Autodesk Inventor part; units mm, degrees
note: some values were not read from the file. Chosen so that the rebuilt part matches the saved one: direction of "Hole2".
(part 12 of 18)
  line L1418 (-102.9071, -28.2921) -> (-102.708, -28.311)
  line L1419 (-102.9072, -28.2921) -> (-102.9071, -28.2921)
  line L1420 (-102.7315, -28.5598) -> (-102.7316, -28.5598)
  line L1421 (-102.708, -28.311) -> (-102.7315, -28.5598)
  line L1422 (-102.8127, -27.2965) -> (-102.8128, -27.2965)
  line L1423 (-102.6136, -27.3154) -> (-102.8127, -27.2965)
  line L1424 (-102.59, -27.0665) -> (-102.6136, -27.3154)
  line L1425 (-102.5901, -27.0665) -> (-102.59, -27.0665)
  line L1426 (-102.9071, -28.2921) -> (-102.8127, -27.2965)
  line L1427 (-102.59, -27.0665) -> (-100.6985, -27.2458)
  line L1428 (-100.84, -28.7391) -> (-102.7315, -28.5598)
  line L1429 (-100.523, -27.5136) -> (-100.6173, -28.5091)
  line L1430 (-100.84, -28.7391) -> (-100.8164, -28.4902)
  line L1431 (-100.8164, -28.4902) -> (-100.6173, -28.5091)
  line L1432 (-100.6173, -28.5091) -> (-100.6174, -28.5091)
  line L1433 (-100.8401, -28.7391) -> (-100.84, -28.7391)
  line L1434 (-100.523, -27.5136) -> (-100.7221, -27.4947)
  line L1435 (-100.7221, -27.4947) -> (-100.6985, -27.2458)
  line L1436 (-102.4145, -27.3343) -> (-100.9212, -27.4758)
  line L1437 (-100.9212, -27.4758) -> (-101.0155, -28.4714)
  line L1438 (-101.0155, -28.4714) -> (-102.5088, -28.3298)
  line L1439 (-102.5088, -28.3298) -> (-102.4145, -27.3343)
  line L1440 (-101.1134, -27.6347) -> (-102.2557, -27.5265)
  line L1441 (-100.9212, -27.4758) -> (-101.1134, -27.6347)
  line L1442 (-102.4145, -27.3343) -> (-102.2557, -27.5265)
  line L1443 (-102.2557, -27.5265) -> (-102.3167, -28.1709)
  line L1444 (-102.5088, -28.3298) -> (-102.3167, -28.1709)
  line L1445 (-102.3167, -28.1709) -> (-101.1745, -28.2792)
  line L1446 (-101.0155, -28.4714) -> (-101.1745, -28.2792)
  line L1447 (-101.1745, -28.2792) -> (-101.1134, -27.6347)
  circle A31 centre (-101.9758, -27.8781) radius 0.1
  line L1448 (-101.8288, -28.0427) -> (-102.1512, -28.0122)
  line L1449 (-102.1512, -28.0122) -> (-102.1228, -27.7135)
  line L1450 (-102.1512, -28.0122) -> (-102.1229, -27.7135)
  line L1451 (-102.1228, -27.7135) -> (-101.8005, -27.7441)
  line L1452 (-101.8005, -27.7441) -> (-101.8288, -28.0427)
  line L1453 (-100.4365, -16.4719) -> (-100.4365, -16.671)
  line L1454 (-100.4365, -16.671) -> (-100.6865, -16.671)
  line L1455 (-99.4365, -16.671) -> (-99.4365, -16.4719)
  line L1456 (-99.1865, -16.671) -> (-99.4365, -16.671)
  line L1457 (-100.4365, -16.4719) -> (-99.4365, -16.4719)
  line L1458 (-99.1865, -16.671) -> (-99.1865, -18.4771)
  line L1459 (-100.6865, -18.4771) -> (-100.6865, -16.671)
  line L1460 (-99.4365, -16.8701) -> (-99.4365, -18.2782)
  line L1461 (-100.4365, -18.2782) -> (-100.4365, -16.8701)
  line L1462 (-100.4365, -16.8701) -> (-99.4365, -16.8701)
  line L1463 (-99.6129, -17.6207) -> (-99.6129, -17.14)
  line L1464 (-99.4365, -16.8701) -> (-99.6129, -17.14)
  line L1465 (-99.6129, -17.14) -> (-100.2602, -17.14)
  line L1466 (-100.4365, -16.8701) -> (-100.2602, -17.14)
  line L1467 (-100.2602, -17.14) -> (-100.2602, -17.6207)
  ellipse E657 centre (-99.9365, -17.4268) end of major axis (-99.8365, -17.4268) minor radius 0.0996
  ellipse E658 centre (-99.9365, -17.4315) end of major axis (-99.8365, -17.4315) minor radius 0.0996 (-100.0365, -17.4315) -> (-99.8365, -17.4315) ccw
  line L1468 (-100.0365, -17.4315) -> (-100.0365, -17.4268)
  line L1469 (-99.8365, -17.4315) -> (-99.8365, -17.4268)
  line L1470 (-100.0865, -17.5927) -> (-100.0865, -17.2703)
  line L1471 (-100.0865, -17.6115) -> (-100.0865, -17.5927)
  line L1472 (-100.0865, -17.2703) -> (-99.7865, -17.2703)
  line L1473 (-99.7865, -17.2703) -> (-99.7865, -17.5927)
  line L1474 (-99.7865, -17.6115) -> (-99.7865, -17.5927)
  line L1475 (-99.7865, -17.5927) -> (-100.0865, -17.5927)
  line L1476 (-99.7865, -17.6115) -> (-100.0865, -17.6115)
  line L1477 (-98.1515, -27.0495) -> (-97.9515, -27.0495)
  line L1478 (-98.1515, -27.08) -> (-98.1515, -27.0495)
  line L1479 (-97.9515, -27.2984) -> (-97.9515, -27.3284)
  line L1480 (-97.9515, -27.0495) -> (-97.9515, -27.2984)
  line L1481 (-97.9515, -26.054) -> (-98.1515, -26.054)
  line L1482 (-97.9515, -25.8051) -> (-97.9515, -26.054)
  line L1483 (-98.1515, -27.0495) -> (-98.1515, -26.054)
  line L1484 (-97.9515, -25.8051) -> (-96.0515, -25.8051)
  line L1485 (-96.0515, -27.2984) -> (-97.9515, -27.2984)
  line L1486 (-95.8515, -26.054) -> (-95.8515, -27.0495)
  line L1487 (-96.0515, -27.2984) -> (-96.0515, -27.0495)
  line L1488 (-96.0515, -27.0495) -> (-95.8515, -27.0495)
  line L1489 (-95.8515, -27.0495) -> (-95.8515, -27.08)
  line L1490 (-96.0515, -27.3284) -> (-96.0515, -27.2984)
  line L1491 (-95.8515, -26.054) -> (-96.0515, -26.054)
  line L1492 (-96.0515, -26.054) -> (-96.0515, -25.8051)
  line L1493 (-97.7515, -26.054) -> (-96.2515, -26.054)
  line L1494 (-96.2515, -26.054) -> (-96.2515, -27.0495)
  line L1495 (-96.2515, -27.0495) -> (-97.7515, -27.0495)
  line L1496 (-97.7515, -27.0495) -> (-97.7515, -26.054)
  line L1497 (-96.2515, -26.054) -> (-96.3121, -26.1467)
  line L1498 (-97.7515, -26.054) -> (-97.691, -26.1467)
  line L1499 (-97.7515, -27.0495) -> (-97.6943, -27.0232)
  line L1500 (-96.2515, -27.0495) -> (-96.3087, -27.0232)
  line L1501 (-93.3858, -28.5091) -> (-93.1866, -28.4902)
  line L1502 (-93.3857, -28.5091) -> (-93.3858, -28.5091)
  line L1503 (-93.1631, -28.7391) -> (-93.163, -28.7391)
  line L1504 (-93.1866, -28.4902) -> (-93.1631, -28.7391)
  line L1505 (-93.281, -27.4947) -> (-93.4801, -27.5136)
  line L1506 (-93.3046, -27.2458) -> (-93.281, -27.4947)
  line L1507 (-93.3858, -28.5091) -> (-93.4801, -27.5136)
  line L1508 (-93.3046, -27.2458) -> (-91.4131, -27.0665)
  line L1509 (-91.2715, -28.5598) -> (-93.1631, -28.7391)
  line L1510 (-91.1904, -27.2965) -> (-91.096, -28.2921)
  line L1511 (-91.4131, -27.0665) -> (-91.413, -27.0665)
  line L1512 (-91.1904, -27.2965) -> (-91.3895, -27.3154)
  line L1513 (-91.3895, -27.3154) -> (-91.4131, -27.0665)
  line L1514 (-91.1903, -27.2965) -> (-91.1904, -27.2965)
  line L1515 (-91.2715, -28.5598) -> (-91.2951, -28.311)
  line L1516 (-91.2951, -28.311) -> (-91.096, -28.2921)
  line L1517 (-91.096, -28.2921) -> (-91.0959, -28.2921)
  line L1518 (-91.2951, -28.311) -> (-91.295, -28.311)
  line L1519 (-91.2714, -28.5598) -> (-91.2715, -28.5598)
  line L1520 (-93.0819, -27.4758) -> (-91.5886, -27.3343)
  line L1521 (-91.5886, -27.3343) -> (-91.4942, -28.3298)
  line L1522 (-91.4942, -28.3298) -> (-92.9875, -28.4714)
  line L1523 (-92.9875, -28.4714) -> (-93.0819, -27.4758)
  line L1524 (-91.7474, -27.5265) -> (-92.8897, -27.6347)
  line L1525 (-91.5886, -27.3343) -> (-91.7474, -27.5265)
  line L1526 (-93.0819, -27.4758) -> (-92.8897, -27.6347)
  line L1527 (-92.8897, -27.6347) -> (-92.8286, -28.2792)
  line L1528 (-92.9875, -28.4714) -> (-92.8286, -28.2792)
  line L1529 (-92.8286, -28.2792) -> (-91.6863, -28.1709)
  line L1530 (-91.4942, -28.3298) -> (-91.6863, -28.1709)
  line L1531 (-91.6863, -28.1709) -> (-91.7474, -27.5265)
  circle A32 centre (-92.5488, -27.9275) radius 0.1
  line L1532 (-92.3734, -28.0616) -> (-92.6958, -28.0922)
  line L1533 (-92.6958, -28.0922) -> (-92.7241, -27.7935)
  line L1534 (-92.7241, -27.7935) -> (-92.4017, -27.7629)
  line L1535 (-92.4017, -27.7629) -> (-92.3734, -28.0616)
  line L1536 (-92.4017, -27.7629) -> (-92.3734, -28.0616)
  line L1537 (-99.5015, -46.2996) -> (-99.5015, -46.0996)
  line L1538 (-99.5015, -46.0996) -> (-99.2515, -46.0996)
  line L1539 (-100.5015, -46.0996) -> (-100.5015, -46.2996)
  line L1540 (-100.7515, -46.0996) -> (-100.5015, -46.0996)
  line L1541 (-99.5015, -46.2996) -> (-100.5015, -46.2996)
  line L1542 (-100.7515, -46.0996) -> (-100.7515, -44.1996)
  line L1543 (-99.2515, -44.1996) -> (-99.2515, -46.0996)
  line L1544 (-100.5015, -43.9996) -> (-99.5015, -43.9996)
  line L1545 (-99.2515, -44.1996) -> (-99.5015, -44.1996)
  line L1546 (-99.5015, -44.1996) -> (-99.5015, -43.9996)
  line L1547 (-100.5015, -43.9996) -> (-100.5015, -44.1996)
  line L1548 (-100.5015, -44.1996) -> (-100.7515, -44.1996)
  line L1549 (-100.5015, -45.8996) -> (-100.5015, -44.3996)
  line L1550 (-100.5015, -44.3996) -> (-99.5015, -44.3996)
  line L1551 (-99.5015, -44.3996) -> (-99.5015, -45.8996)
  line L1552 (-99.5015, -45.8996) -> (-100.5015, -45.8996)
  line L1553 (-100.3252, -44.5759) -> (-100.3252, -45.7232)
  line L1554 (-100.5015, -44.3996) -> (-100.3252, -44.5759)
  line L1555 (-100.5015, -45.8996) -> (-100.3252, -45.7232)
  line L1556 (-100.3252, -45.7232) -> (-99.6779, -45.7232)
  line L1557 (-99.5015, -45.8996) -> (-99.6779, -45.7232)
  line L1558 (-99.6779, -45.7232) -> (-99.6779, -44.5759)
  line L1559 (-99.5015, -44.3996) -> (-99.6779, -44.5759)
  line L1560 (-99.6779, -44.5759) -> (-100.3252, -44.5759)
  circle A33 centre (-100.0015, -45.4115) radius 0.1
  line L1561 (-99.8515, -45.2496) -> (-99.8515, -45.5734)
  line L1562 (-99.8515, -45.5734) -> (-100.1515, -45.5734)
  line L1563 (-100.1515, -45.5734) -> (-100.1515, -45.2496)
  line L1564 (-100.1515, -45.2496) -> (-99.8515, -45.2496)
  line L1565 (-95.8515, -35.7016) -> (-96.0515, -35.7016)
  line L1566 (-96.0515, -35.7016) -> (-96.0515, -35.4516)
  line L1567 (-96.0515, -36.7016) -> (-95.8515, -36.7016)
  line L1568 (-96.0515, -36.9516) -> (-96.0515, -36.7016)
  line L1569 (-95.8515, -35.7016) -> (-95.8515, -36.7016)
  line L1570 (-96.0515, -36.9516) -> (-97.9515, -36.9516)
  line L1571 (-97.9515, -35.4516) -> (-96.0515, -35.4516)
  line L1572 (-98.1515, -36.7016) -> (-98.1515, -35.7016)
  line L1573 (-97.9515, -35.4516) -> (-97.9515, -35.7016)
  line L1574 (-97.9515, -35.7016) -> (-98.1515, -35.7016)
  line L1575 (-98.1515, -36.7016) -> (-97.9515, -36.7016)
  line L1576 (-97.9515, -36.7016) -> (-97.9515, -36.9516)
  line L1577 (-96.2515, -36.7016) -> (-97.7515, -36.7016)
  line L1578 (-97.7515, -36.7016) -> (-97.7515, -35.7016)
  line L1579 (-97.7515, -35.7016) -> (-96.2515, -35.7016)
  line L1580 (-96.2515, -35.7016) -> (-96.2515, -36.7016)
  line L1581 (-97.5752, -36.5252) -> (-96.4279, -36.5252)
  line L1582 (-97.7515, -36.7016) -> (-97.5752, -36.5252)
  line L1583 (-96.2515, -36.7016) -> (-96.4279, -36.5252)
  line L1584 (-96.4279, -36.5252) -> (-96.4279, -35.8779)
  line L1585 (-96.2515, -35.7016) -> (-96.4279, -35.8779)
  line L1586 (-96.4279, -35.8779) -> (-97.5752, -35.8779)
  line L1587 (-97.7515, -35.7016) -> (-97.5752, -35.8779)
  line L1588 (-97.5752, -35.8779) -> (-97.5752, -36.5252)
  circle A34 centre (-96.7396, -36.2016) radius 0.1
  line L1589 (-96.9015, -36.0516) -> (-96.5777, -36.0516)
  line L1590 (-96.5777, -36.0516) -> (-96.5777, -36.3516)
  line L1591 (-96.5777, -36.3516) -> (-96.9015, -36.3516)
  line L1592 (-96.9015, -36.3516) -> (-96.9015, -36.0516)
  line L1593 (-93.5015, -46.2996) -> (-93.5015, -46.0996)
  line L1594 (-93.5015, -46.0996) -> (-93.2515, -46.0996)
  line L1595 (-94.5015, -46.0996) -> (-94.5015, -46.2996)
  line L1596 (-94.7515, -46.0996) -> (-94.5015, -46.0996)
  line L1597 (-93.5015, -46.2996) -> (-94.5015, -46.2996)
  line L1598 (-94.7515, -46.0996) -> (-94.7515, -44.1996)
  line L1599 (-93.2515, -44.1996) -> (-93.2515, -46.0996)
  line L1600 (-94.5015, -43.9996) -> (-93.5015, -43.9996)
  line L1601 (-93.2515, -44.1996) -> (-93.5015, -44.1996)
  line L1602 (-93.5015, -44.1996) -> (-93.5015, -43.9996)
  line L1603 (-94.5015, -43.9996) -> (-94.5015, -44.1996)
  line L1604 (-94.5015, -44.1996) -> (-94.7515, -44.1996)
  line L1605 (-94.5015, -45.8996) -> (-94.5015, -44.3996)
  line L1606 (-94.5015, -44.3996) -> (-93.5015, -44.3996)
  line L1607 (-93.5015, -44.3996) -> (-93.5015, -45.8996)
  line L1608 (-93.5015, -45.8996) -> (-94.5015, -45.8996)
  line L1609 (-94.3252, -44.5759) -> (-94.3252, -45.7232)
  line L1610 (-94.5015, -44.3996) -> (-94.3252, -44.5759)
  line L1611 (-94.5015, -45.8996) -> (-94.3252, -45.7232)
  line L1612 (-94.3252, -45.7232) -> (-93.6779, -45.7232)
  line L1613 (-93.5015, -45.8996) -> (-93.6779, -45.7232)
  line L1614 (-93.6779, -45.7232) -> (-93.6779, -44.5759)
  line L1615 (-93.5015, -44.3996) -> (-93.6779, -44.5759)
  line L1616 (-93.6779, -44.5759) -> (-94.3252, -44.5759)
  circle A35 centre (-94.0015, -45.4115) radius 0.1
  line L1617 (-93.8515, -45.2496) -> (-93.8515, -45.5734)
  line L1618 (-93.8515, -45.5734) -> (-94.1515, -45.5734)
  line L1619 (-94.1515, -45.5734) -> (-94.1515, -45.2496)
  line L1620 (-94.1515, -45.2496) -> (-93.8515, -45.2496)
  line L1621 (-93.5665, -18.2782) -> (-93.5665, -18.4771)
  line L1622 (-93.5665, -18.4771) -> (-93.3165, -18.4771)
  line L1623 (-94.5665, -18.4771) -> (-94.5665, -18.2782)
  line L1624 (-94.8165, -18.4771) -> (-94.5665, -18.4771)
  line L1625 (-93.5665, -18.2782) -> (-94.5665, -18.2782)
  line L1626 (-94.8165, -18.4771) -> (-94.8165, -20.235)
  line L1627 (-93.3165, -20.235) -> (-93.3165, -18.4771)
  line L1628 (-94.5665, -18.676) -> (-94.5665, -20.0364)
  line L1629 (-93.5665, -18.676) -> (-94.5665, -18.676)
  line L1630 (-93.5665, -20.0364) -> (-93.5665, -18.676)
  line L1631 (-94.5665, -18.676) -> (-94.4066, -18.9295)
  line L1632 (-93.5665, -18.676) -> (-93.7265, -18.9295)
  ellipse E659 centre (-94.0665, -19.2395) end of major axis (-94.1665, -19.2395) minor radius 0.0995
  ellipse E660 centre (-94.0665, -19.2447) end of major axis (-94.1665, -19.2447) minor radius 0.0995 (-94.1665, -19.2447) -> (-93.9665, -19.2447) ccw
  line L1633 (-93.9665, -19.2395) -> (-93.9665, -19.2447)
  line L1634 (-94.1665, -19.2395) -> (-94.1665, -19.2447)
  line L1635 (-93.9165, -19.4057) -> (-93.9165, -19.0837)
  line L1636 (-93.9165, -19.4163) -> (-93.9165, -19.4057)
  line L1637 (-93.9165, -19.0837) -> (-94.2165, -19.0837)
  line L1638 (-94.2165, -19.0837) -> (-94.2165, -19.4057)
  line L1639 (-94.2165, -19.4163) -> (-94.2165, -19.4057)
  line L1640 (-94.2165, -19.4057) -> (-93.9165, -19.4057)
  line L1641 (-89.2199, -19.61) -> (-89.2407, -19.4112)
  line L1642 (-89.2407, -19.4112) -> (-89.2409, -19.4111)
  line L1643 (-89.2409, -19.4111) -> (-89.2201, -19.6101)
  line L1644 (-89.2201, -19.6101) -> (-88.9715, -19.584)
  line L1645 (-88.9715, -19.584) -> (-88.9712, -19.5841)
  line L1646 (-90.2147, -19.7141) -> (-90.2355, -19.5152)
  line L1647 (-90.4633, -19.7401) -> (-90.2147, -19.7141)
  line L1648 (-88.7887, -21.3283) -> (-88.9712, -19.5841)
  line L1649 (-89.9959, -21.8028) -> (-89.7318, -21.7752)
  line L1650 (-89.2409, -19.4111) -> (-90.2355, -19.5152)
  line L1651 (-90.4633, -19.7401) -> (-90.2656, -21.6298)
  line L1652 (-89.9962, -21.8027) -> (-89.0016, -21.6987)
  line L1653 (-88.7738, -21.4737) -> (-88.9715, -19.584)
  line L1654 (-90.2654, -21.6299) -> (-90.017, -21.6039)
  line L1655 (-90.2656, -21.6298) -> (-90.2654, -21.6299)
  line L1656 (-90.017, -21.6038) -> (-90.2656, -21.6298)
  line L1657 (-89.9962, -21.8027) -> (-90.017, -21.6038)
  line L1658 (-89.9959, -21.8028) -> (-89.9962, -21.8027)
  line L1659 (-89.0224, -21.4997) -> (-89.0016, -21.6987)
  line L1660 (-88.7738, -21.4737) -> (-89.0224, -21.4997)
  line L1661 (-90.1939, -19.913) -> (-90.0378, -21.4049)
  line L1662 (-89.1993, -19.809) -> (-90.1939, -19.913)
  line L1663 (-89.0432, -21.3008) -> (-89.1993, -19.809)
  line L1664 (-90.0378, -21.4049) -> (-89.0432, -21.3008)
  line L1665 (-89.8806, -21.2112) -> (-90, -20.0701)
  line L1666 (-90.1939, -19.913) -> (-90, -20.0701)
  line L1667 (-90.0378, -21.4049) -> (-89.8806, -21.2112)
  line L1668 (-90, -20.0701) -> (-89.3562, -20.0027)
  line L1669 (-89.1993, -19.809) -> (-89.3562, -20.0027)
  line L1670 (-89.3562, -20.0027) -> (-89.2368, -21.1439)
  line L1671 (-89.0432, -21.3008) -> (-89.2368, -21.1439)
  line L1672 (-89.2368, -21.1439) -> (-89.8806, -21.2112)
  circle A36 centre (-89.6457, -20.3465) radius 0.1
  line L1673 (-89.4796, -20.4919) -> (-89.5133, -20.1698)
  line L1674 (-89.4796, -20.4919) -> (-89.4796, -20.4919)
  line L1675 (-89.4796, -20.4919) -> (-89.5133, -20.1698)
  line L1676 (-89.5133, -20.1698) -> (-89.5133, -20.1698)
  line L1677 (-89.5133, -20.1698) -> (-89.8117, -20.2011)
  line L1678 (-89.8117, -20.2011) -> (-89.778, -20.5231)
  line L1679 (-89.778, -20.5231) -> (-89.778, -20.5231)
  line L1680 (-89.778, -20.5231) -> (-89.4796, -20.4919)
  line L1681 (-89.778, -20.5231) -> (-89.4796, -20.4919)
  line L1682 (-93.5665, -20.0364) -> (-93.5665, -20.235)
  line L1683 (-93.5665, -20.235) -> (-93.3165, -20.235)
  line L1684 (-94.5665, -20.235) -> (-94.5665, -20.0364)
  line L1685 (-94.8165, -20.235) -> (-94.5665, -20.235)
  line L1686 (-93.5665, -22.2845) -> (-93.3165, -22.2845)
  line L1687 (-93.5665, -22.1222) -> (-93.5665, -22.3209)
  line L1688 (-93.3165, -22.1222) -> (-93.5665, -22.1222)
  line L1689 (-93.5665, -22.3209) -> (-93.5665, -22.4832)
  line L1690 (-93.3165, -22.2845) -> (-93.3165, -22.1222)
  line L1691 (-94.5665, -22.4832) -> (-93.5665, -22.4832)
  line L1692 (-93.5665, -20.0364) -> (-94.5665, -20.0364)
  line L1693 (-94.8165, -20.235) -> (-94.8165, -22.1222)
  line L1694 (-94.5665, -22.3209) -> (-93.5665, -22.3209)
  line L1695 (-93.3165, -22.1222) -> (-93.3165, -20.235)
  line L1696 (-94.8165, -22.2845) -> (-94.5665, -22.2845)
  line L1697 (-94.8165, -22.1222) -> (-94.8165, -22.2845)
  line L1698 (-94.5665, -22.1222) -> (-94.8165, -22.1222)
  line L1699 (-94.5665, -22.3209) -> (-94.5665, -22.1222)
  line L1700 (-94.5665, -22.4832) -> (-94.5665, -22.3209)
  line L1701 (-94.5665, -20.4337) -> (-94.5665, -21.9236)
  line L1702 (-93.5665, -20.4337) -> (-94.5665, -20.4337)
  line L1703 (-93.5665, -21.9236) -> (-93.5665, -20.4337)
  line L1704 (-94.5665, -21.9236) -> (-93.5665, -21.9236)
  line L1705 (-94.3902, -21.8644) -> (-94.3902, -20.7247)
  line L1706 (-94.5665, -20.4337) -> (-94.3902, -20.7247)
  line L1707 (-94.5665, -21.9236) -> (-94.3902, -21.8644)
  line L1708 (-94.3902, -20.7247) -> (-93.7429, -20.7247)
  line L1709 (-93.5665, -20.4337) -> (-93.7429, -20.7247)
  line L1710 (-93.7429, -20.7247) -> (-93.7429, -21.8644)
  line L1711 (-93.5665, -21.9236) -> (-93.7429, -21.8644)
  line L1712 (-93.7429, -21.8644) -> (-94.3902, -21.8644)
  ellipse E661 centre (-94.0665, -21.0054) end of major axis (-94.1665, -21.0054) minor radius 0.0993
  ellipse E662 centre (-94.0665, -21.0112) end of major axis (-94.1665, -21.0112) minor radius 0.0993 (-94.1665, -21.0112) -> (-93.9665, -21.0112) ccw
  line L1713 (-93.9665, -21.0054) -> (-93.9665, -21.0112)
  line L1714 (-94.1665, -21.0054) -> (-94.1665, -21.0112)
  line L1715 (-93.9165, -21.172) -> (-93.9165, -20.8504)
  line L1716 (-93.9165, -21.1952) -> (-93.9165, -21.172)
  line L1717 (-93.9165, -20.8504) -> (-94.2165, -20.8504)
  line L1718 (-94.2165, -20.8504) -> (-94.2165, -21.172)
  line L1719 (-94.2165, -21.1952) -> (-94.2165, -21.172)
  line L1720 (-94.2165, -21.172) -> (-93.9165, -21.172)
  line L1721 (-94.2165, -21.1952) -> (-93.9165, -21.1952)
  line L1722 (-88.5289, -21.2981) -> (-88.529, -21.298)
  line L1723 (-88.529, -21.298) -> (-88.5058, -21.4966)
  line L1724 (-88.5058, -21.4966) -> (-88.2575, -21.4676)
  line L1725 (-88.2575, -21.4676) -> (-88.2574, -21.4677)
  line L1726 (-88.0369, -23.3549) -> (-88.2574, -21.4677)
  line L1727 (-88.2896, -23.5857) -> (-88.262, -23.5825)
  line L1728 (-88.529, -21.298) -> (-88.789, -21.3284)
  line L1729 (-89.7318, -21.7751) -> (-89.5269, -23.5289)
  line L1730 (-89.2554, -23.6985) -> (-88.2621, -23.5825)
  line L1731 (-88.037, -23.3548) -> (-88.2575, -21.4676)
  line L1732 (-88.2573, -23.3806) -> (-88.0369, -23.3549)
  line L1733 (-88.262, -23.5825) -> (-88.2733, -23.4858)
  line L1734 (-88.2853, -23.3838) -> (-88.2621, -23.5825)
  line L1735 (-88.037, -23.3548) -> (-88.2853, -23.3838)
  line L1736 (-88.2853, -23.3838) -> (-88.2852, -23.3839)
  line L1737 (-88.2621, -23.5825) -> (-88.262, -23.5825)
  line L1738 (-88.0369, -23.3549) -> (-88.037, -23.3548)
  line L1739 (-89.5269, -23.5289) -> (-89.5267, -23.5289)
  line L1740 (-89.2786, -23.4999) -> (-89.5269, -23.5289)
  line L1741 (-89.2554, -23.6985) -> (-89.2786, -23.4999)
  line L1742 (-89.2552, -23.6986) -> (-89.2554, -23.6985)
  line L1743 (-89.4758, -21.8113) -> (-89.3018, -23.3012)
  line L1744 (-88.4826, -21.6953) -> (-89.4758, -21.8113)
  line L1745 (-88.3085, -23.1852) -> (-88.4826, -21.6953)
  line L1746 (-89.3018, -23.3012) -> (-88.3085, -23.1852)
  line L1747 (-89.147, -23.1057) -> (-89.2801, -21.9661)
  line L1748 (-89.4758, -21.8113) -> (-89.2801, -21.9661)
  line L1749 (-89.3018, -23.3012) -> (-89.147, -23.1057)
  line L1750 (-89.2801, -21.9661) -> (-88.6372, -21.8909)
  line L1751 (-88.4826, -21.6953) -> (-88.6372, -21.8909)
  line L1752 (-88.6372, -21.8909) -> (-88.504, -23.0305)
  line L1753 (-88.3085, -23.1852) -> (-88.504, -23.0305)
  line L1754 (-88.504, -23.0305) -> (-89.147, -23.1057)
  circle A37 centre (-88.9225, -22.2381) radius 0.1
  line L1755 (-88.7547, -22.3816) -> (-88.7923, -22.0599)
  line L1756 (-88.7547, -22.3816) -> (-88.7547, -22.3816)
  line L1757 (-88.7547, -22.3816) -> (-88.7923, -22.0599)
  line L1758 (-88.7923, -22.0599) -> (-88.7923, -22.0599)
  line L1759 (-88.7923, -22.0599) -> (-89.0903, -22.0947)
  line L1760 (-89.0903, -22.0947) -> (-89.0527, -22.4164)
  line L1761 (-89.0527, -22.4164) -> (-89.0527, -22.4164)
  line L1762 (-89.0527, -22.4164) -> (-88.7547, -22.3816)
  line L1763 (-89.0527, -22.4164) -> (-88.7547, -22.3816)
  line L1764 (-93.5665, -16.4719) -> (-93.5665, -16.671)
  line L1765 (-93.5665, -16.671) -> (-93.3165, -16.671)
  line L1766 (-94.5665, -16.671) -> (-94.5665, -16.4719)
  line L1767 (-94.8165, -16.671) -> (-94.5665, -16.671)
  line L1768 (-93.5665, -16.4719) -> (-94.5665, -16.4719)
  line L1769 (-94.8165, -16.671) -> (-94.8165, -18.4771)
  line L1770 (-93.3165, -18.4771) -> (-93.3165, -16.671)
  line L1771 (-94.5665, -16.8701) -> (-94.5665, -18.2782)
  line L1772 (-93.5665, -16.8701) -> (-94.5665, -16.8701)
  line L1773 (-93.5665, -18.2782) -> (-93.5665, -16.8701)
  line L1774 (-94.3902, -17.6207) -> (-94.3902, -17.14)
  line L1775 (-94.5665, -16.8701) -> (-94.3902, -17.14)
  line L1776 (-94.3902, -17.14) -> (-93.7429, -17.14)
  line L1777 (-93.5665, -16.8701) -> (-93.7429, -17.14)
  line L1778 (-93.7429, -17.14) -> (-93.7429, -17.6207)
  ellipse E663 centre (-94.0665, -17.4268) end of major axis (-94.1665, -17.4268) minor radius 0.0996
  ellipse E664 centre (-94.0665, -17.4315) end of major axis (-94.1665, -17.4315) minor radius 0.0996 (-94.1665, -17.4315) -> (-93.9665, -17.4315) ccw
  line L1779 (-93.9665, -17.4268) -> (-93.9665, -17.4315)
  line L1780 (-94.1665, -17.4268) -> (-94.1665, -17.4315)
  line L1781 (-93.9165, -17.5927) -> (-93.9165, -17.2703)
  line L1782 (-93.9165, -17.6115) -> (-93.9165, -17.5927)
  line L1783 (-93.9165, -17.2703) -> (-94.2165, -17.2703)
  line L1784 (-94.2165, -17.2703) -> (-94.2165, -17.5927)
  line L1785 (-94.2165, -17.6115) -> (-94.2165, -17.5927)
  line L1786 (-94.2165, -17.5927) -> (-93.9165, -17.5927)
  line L1787 (-94.2165, -17.6115) -> (-93.9165, -17.6115)
  line L1788 (-89.8049, -17.698) -> (-89.8237, -17.4989)
  line L1789 (-89.8237, -17.4989) -> (-89.8238, -17.4989)
  line L1790 (-89.8238, -17.4989) -> (-89.805, -17.698)
  line L1791 (-89.805, -17.698) -> (-89.5561, -17.6744)
  line L1792 (-89.5561, -17.6744) -> (-89.556, -17.6744)
  line L1793 (-90.8005, -17.7923) -> (-90.8194, -17.5932)
  line L1794 (-91.0494, -17.8159) -> (-90.8005, -17.7923)
  line L1795 (-89.5351, -17.8945) -> (-89.556, -17.6744)
  line L1796 (-89.8238, -17.4989) -> (-90.8194, -17.5932)
  line L1797 (-91.0494, -17.8159) -> (-90.8701, -19.7075)
  line L1798 (-90.6023, -19.883) -> (-90.4499, -19.8685)
  line L1799 (-89.39, -19.4267) -> (-89.5561, -17.6744)
  line L1800 (-90.8701, -19.7075) -> (-90.87, -19.7075)
  line L1801 (-90.6212, -19.6839) -> (-90.8701, -19.7075)
  line L1802 (-90.6023, -19.883) -> (-90.6212, -19.6839)
  line L1803 (-90.6022, -19.883) -> (-90.6023, -19.883)
  line L1804 (-90.7816, -17.9914) -> (-90.6401, -19.4848)
  line L1805 (-89.7861, -17.8971) -> (-90.7816, -17.9914)
  line L1806 (-89.6445, -19.3904) -> (-89.7861, -17.8971)
  line L1807 (-90.6401, -19.4848) -> (-89.6445, -19.3904)
  line L1808 (-90.4811, -19.2926) -> (-90.5894, -18.1504)
  line L1809 (-90.7816, -17.9914) -> (-90.5894, -18.1504)
  line L1810 (-90.6401, -19.4848) -> (-90.4811, -19.2926)
  line L1811 (-90.5894, -18.1504) -> (-89.9449, -18.0893)
  line L1812 (-89.7861, -17.8971) -> (-89.9449, -18.0893)
  line L1813 (-89.9449, -18.0893) -> (-89.8366, -19.2315)
  line L1814 (-89.6445, -19.3904) -> (-89.8366, -19.2315)
  line L1815 (-89.8366, -19.2315) -> (-90.4811, -19.2926)
  circle A38 centre (-90.2377, -18.4302) radius 0.1
  line L1816 (-90.0731, -18.5772) -> (-90.1037, -18.2548)
  line L1817 (-90.0731, -18.5772) -> (-90.1037, -18.2548)
  line L1818 (-90.1037, -18.2548) -> (-90.4023, -18.2831)
  line L1819 (-90.4023, -18.2831) -> (-90.3718, -18.6055)
  line L1820 (-90.3718, -18.6055) -> (-90.0731, -18.5772)
  ellipse E665 centre (-107.527, -21.5715) end of major axis (-108.7255, -21.632) minor radius 0.2145 (-106.7704, -21.3679) -> (-108.7036, -21.6699) ccw
  ellipse E666 centre (-107.5171, -21.768) end of major axis (-108.5158, -21.8185) minor radius 0.1787 (-106.985, -21.5905) -> (-108.3033, -21.9168) ccw
  line L1821 (-108.4975, -21.8501) -> (-108.7036, -21.6699)
  ellipse E667 centre (-107.5171, -21.768) end of major axis (-108.2661, -21.8059) minor radius 0.134 (-107.2416, -21.6297) -> (-108.0565, -21.8875) ccw
  line L1822 (-108.7255, -21.632) -> (-108.7684, -20.7835)
  ellipse E668 centre (-86.4761, -21.5715) end of major axis (-85.2776, -21.632) minor radius 0.2145 (-85.2995, -21.6699) -> (-87.2327, -21.3679) ccw
  ellipse E669 centre (-86.486, -21.768) end of major axis (-85.4873, -21.8185) minor radius 0.1787 (-85.6997, -21.9168) -> (-87.018, -21.5905) ccw
  line L1823 (-85.5055, -21.8501) -> (-85.2995, -21.6699)
  ellipse E670 centre (-86.486, -21.768) end of major axis (-85.737, -21.8059) minor radius 0.134 (-85.9466, -21.8875) -> (-86.7615, -21.6297) ccw
  line L1824 (-85.2776, -21.632) -> (-85.2347, -20.7835)
  ellipse E671 centre (-97.0015, -6.8845) end of major axis (-97.568, -6.8845) minor radius 0.5639 (-96.6326, -7.3123) -> (-97.3705, -7.3123) ccw
  line L1825 (-97.1151, -6.4917) -> (-96.7166, -6.5901)
  line L1826 (-96.7166, -6.5901) -> (-96.603, -6.983)
  line L1827 (-96.603, -6.983) -> (-96.8647, -7.2534)
  line L1828 (-97.1163, -7.2209) -> (-97.2865, -7.1789)
  line L1829 (-97.2865, -7.1789) -> (-97.4001, -6.786)
  line L1830 (-97.4001, -6.786) -> (-97.1151, -6.4917)
  line L1831 (-96.7166, -6.5901) -> (-96.7166, -6.6798)
  line L1832 (-97.1151, -6.5809) -> (-97.1151, -6.4917)
  spline S82 degree 3 poles (-108.5966, -51.7047) (-108.5918, -51.7053) (-108.5815, -51.7066) (-108.5668, -51.7163) (-108.5523, -51.7308) (-108.5379, -51.7511) (-108.524, -51.7768) (-108.5054, -51.8196) (-108.4896, -51.8686) (-108.476, -51.9231) (-108.4626, -51.9874) (-108.4493, -52.0758) (-108.4399, -52.187) (-108.4366, -52.3016) (-108.4399, -52.4161) (-108.4493, -52.5274) (-108.4626, -52.6157) (-108.476, -52.68) (-108.4896, -52.7345) (-108.5054, -52.7836) (-108.524, -52.8263) (-108.5379, -52.852) (-108.5523, -52.8723) (-108.5668, -52.8868) (-108.5815, -52.8965) (-108.5918, -52.8978) (-108.5966, -52.8985) knots 0 0 0 0 0.011067 0.024078 0.039928 0.05914 0.081934 0.10802 0.168059 0.202015 0.239296 0.321668 0.410563 0.5 0.589437 0.678332 0.760704 0.797985 0.831941 0.89198 0.918066 0.94086 0.960072 0.975922 0.988933 1 1 1 1
  spline S83 degree 3 poles (-108.5966, -52.8985) (-108.6012, -52.8979) (-108.6113, -52.8965) (-108.6252, -52.8869) (-108.6384, -52.8723) (-108.6509, -52.8519) (-108.6626, -52.8262) (-108.6777, -52.7833) (-108.6898, -52.7343) (-108.6998, -52.68) (-108.7095, -52.6155) (-108.7187, -52.5272) (-108.725, -52.416) (-108.7272, -52.3016) (-108.725, -52.1871) (-108.7187, -52.076) (-108.7095, -51.9876) (-108.6998, -51.9232) (-108.6898, -51.8688) (-108.6777, -51.8198) (-108.6626, -51.7769) (-108.6509, -51.7512) (-108.6384, -51.7309) (-108.6252, -51.7163) (-108.6113, -51.7066) (-108.6012, -51.7053) (-108.5966, -51.7047) knots 0 0 0 0 0.010997 0.023628 0.038954 0.057614 0.079908 0.105595 0.165209 0.199149 0.236543 0.319515 0.409403 0.5 0.590597 0.680485 0.763457 0.800851 0.834791 0.894405 0.920092 0.942386 0.961046 0.976372 0.989003 1 1 1 1
  spline S84 degree 3 poles (-85.4065, -52.8985) (-85.4113, -52.8978) (-85.4216, -52.8965) (-85.4362, -52.8868) (-85.4508, -52.8723) (-85.4652, -52.852) (-85.4791, -52.8263) (-85.4977, -52.7836) (-85.5135, -52.7345) (-85.5271, -52.68) (-85.5405, -52.6157) (-85.5538, -52.5274) (-85.5632, -52.4161) (-85.5665, -52.3016) (-85.5632, -52.187) (-85.5538, -52.0758) (-85.5405, -51.9874) (-85.5271, -51.9231) (-85.5135, -51.8686) (-85.4977, -51.8196) (-85.4791, -51.7768) (-85.4652, -51.7511) (-85.4508, -51.7308) (-85.4362, -51.7163) (-85.4216, -51.7066) (-85.4113, -51.7053) (-85.4065, -51.7047) knots 0 0 0 0 0.011067 0.024078 0.039928 0.05914 0.081934 0.10802 0.168059 0.202015 0.239296 0.321668 0.410563 0.5 0.589437 0.678332 0.760704 0.797985 0.831941 0.89198 0.918066 0.94086 0.960072 0.975922 0.988933 1 1 1 1
  spline S85 degree 3 poles (-85.4065, -51.7047) (-85.4018, -51.7053) (-85.3918, -51.7066) (-85.3779, -51.7163) (-85.3647, -51.7309) (-85.3521, -51.7512) (-85.3405, -51.7769) (-85.3254, -51.8198) (-85.3133, -51.8688) (-85.3033, -51.9232) (-85.2936, -51.9876) (-85.2843, -52.076) (-85.278, -52.1871) (-85.2758, -52.3016) (-85.278, -52.416) (-85.2843, -52.5272) (-85.2936, -52.6155) (-85.3033, -52.68) (-85.3133, -52.7343) (-85.3254, -52.7833) (-85.3405, -52.8262) (-85.3521, -52.8519) (-85.3647, -52.8723) (-85.3779, -52.8869) (-85.3918, -52.8965) (-85.4018, -52.8979) (-85.4065, -52.8985) knots 0 0 0 0 0.010997 0.023628 0.038954 0.057614 0.079908 0.105595 0.165209 0.199149 0.236543 0.319515 0.409403 0.5 0.590597 0.680485 0.763457 0.800851 0.834791 0.894405 0.920092 0.942386 0.961046 0.976372 0.989003 1 1 1 1
  line L1833 (-101.2148, -54.7096) -> (-101.2148, -54.8016)
  line L1834 (-106.1558, -54.8016) -> (-106.1558, -54.2016)
  line L1835 (-101.2148, -54.8016) -> (-106.1558, -54.8016)
  line L1836 (-92.7883, -54.8016) -> (-92.7883, -54.7096)
  line L1837 (-87.8473, -54.8016) -> (-92.7883, -54.8016)
  line L1838 (-87.8473, -54.2016) -> (-87.8473, -54.8016)
  line L1839 (-101.0015, -54.2016) -> (-106.1558, -54.2016)
  line L1840 (-87.8473, -54.2016) -> (-93.0015, -54.2016)
  line L1841 (-85.0515, -54.8016) -> (-87.8473, -54.8016)
  line L1842 (-106.1558, -54.8016) -> (-108.9515, -54.8016)
  line L1843 (-93.0015, -49.8016) -> (-85.0515, -49.8016)
  line L1844 (-108.9515, -49.8016) -> (-101.0015, -49.8016)
  line L1845 (-108.9515, -54.8016) -> (-108.9515, -49.8016)
  line L1846 (-85.0515, -54.8016) -> (-85.0515, -49.8016)
  line L1847 (-92.7883, -54.8016) -> (-93.0982, -54.8016)
  line L1848 (-93.0982, -54.8016) -> (-93.0982, -54.7096)
  line L1849 (-93.0982, -54.8016) -> (-101.2148, -54.8016)
  line L1850 (-106.0839, -39.8016) -> (-100.3267, -39.8016)
  line L1851 (-93.6764, -39.8016) -> (-87.9192, -39.8016)
  line L1852 (-86.3513, -39.8016) -> (-85.7882, -39.8016)
  line L1853 (-108.2148, -39.8016) -> (-107.6518, -39.8016)
  line L1854 (-85.7882, -49.8016) -> (-85.7882, -39.8016)
  line L1855 (-108.2148, -39.8016) -> (-108.2148, -49.8016)
  spline S86 degree 3 poles (-105.7693, -47.2006) (-105.7691, -47.0904) (-105.7657, -46.8664) (-105.7476, -46.534) (-105.7174, -46.2608) (-105.6841, -46.0715) (-105.6496, -45.9793) (-105.6262, -45.9168) (-105.577, -45.9143) (-105.5494, -45.9544) (-105.5145, -46.035) (-105.4774, -46.2212) (-105.4459, -46.4945) (-105.428, -46.826) (-105.4236, -47.1593) (-105.4311, -47.4922) (-105.4511, -47.8261) (-105.483, -48.0981) (-105.5188, -48.2878) (-105.5513, -48.3791) (-105.5751, -48.4448) (-105.6244, -48.445) (-105.6508, -48.4035) (-105.6816, -48.3228) (-105.7187, -48.1371) (-105.7479, -47.8647) (-105.7654, -47.5325) (-105.7696, -47.3099) (-105.7693, -47.2006) knots 0 0 0 0 0.063707 0.129495 0.191912 0.223688 0.23829 0.25135 0.256604 0.263018 0.277149 0.308538 0.37104 0.436878 0.500023 0.563695 0.629383 0.692836 0.723161 0.738573 0.75181 0.756962 0.76326 0.777952 0.808043 0.871314 0.936843 1 1 1 1
  spline S87 degree 3 poles (-107.9655, -47.119) (-107.9649, -46.8963) (-107.9545, -46.5724) (-107.9545, -46.176) (-107.9167, -46.0179) (-107.926, -45.9241) (-107.8893, -45.9141) (-107.8786, -45.9945) (-107.8601, -46.0819) (-107.845, -46.3022) (-107.8316, -46.572) (-107.8242, -46.9058) (-107.8202, -47.3522) (-107.8358, -47.7851) (-107.8394, -48.1822) (-107.8791, -48.3411) (-107.8698, -48.4357) (-107.9071, -48.4462) (-107.9157, -48.3637) (-107.9337, -48.2767) (-107.946, -48.0556) (-107.962, -47.6783) (-107.9661, -47.342) (-107.9655, -47.119) knots 0 0 0 0 0.131392 0.195062 0.224866 0.236537 0.238771 0.243638 0.272647 0.302988 0.368078 0.435032 0.499113 0.631038 0.694715 0.724747 0.73665 0.738894 0.743873 0.773079 0.803452 0.868455 1 1 1 1
  spline S88 degree 3 poles (-88.5776, -47.119) (-88.5773, -47.0087) (-88.5742, -46.7841) (-88.5524, -46.4552) (-88.5229, -46.1745) (-88.4755, -46.0079) (-88.4394, -45.9161) (-88.3904, -45.9148) (-88.3471, -45.977) (-88.3166, -46.088) (-88.2798, -46.3002) (-88.2526, -46.5763) (-88.2362, -46.9076) (-88.232, -47.2409) (-88.239, -47.5743) (-88.2586, -47.9035) (-88.2891, -48.183) (-88.3328, -48.3506) (-88.3651, -48.4425) (-88.4146, -48.4462) (-88.4582, -48.3807) (-88.486, -48.2716) (-88.5273, -48.0592) (-88.5545, -47.7842) (-88.5736, -47.4511) (-88.5779, -47.2282) (-88.5776, -47.119) knots 0 0 0 0 0.063774 0.129476 0.191917 0.222516 0.235727 0.240982 0.247121 0.27643 0.308417 0.371002 0.43691 0.500019 0.563738 0.62925 0.691939 0.722123 0.735387 0.74054 0.746943 0.777028 0.807219 0.871188 0.93687 1 1 1 1
  line L1856 (-87.9192, -39.8016) -> (-86.3513, -39.8016)
  line L1857 (-107.6518, -39.8016) -> (-106.0839, -39.8016)
  spline S89 degree 3 poles (-86.1803, -47.2006) (-86.1796, -46.9767) (-86.1777, -46.6427) (-86.1534, -46.2637) (-86.1447, -46.0707) (-86.1211, -45.9854) (-86.1276, -45.9196) (-86.0903, -45.9162) (-86.0868, -45.9616) (-86.0674, -46.0338) (-86.0586, -46.2256) (-86.0441, -46.4942) (-86.0385, -46.8265) (-86.0367, -47.272) (-86.0401, -47.7177) (-86.0612, -48.0946) (-86.0686, -48.2894) (-86.0901, -48.3717) (-86.0826, -48.4434) (-86.1202, -48.4425) (-86.1233, -48.3969) (-86.1429, -48.324) (-86.1544, -48.1332) (-86.177, -47.7572) (-86.181, -47.4231) (-86.1803, -47.2006) knots 0 0 0 0 0.132092 0.195475 0.227359 0.241584 0.252969 0.255186 0.260256 0.27356 0.304855 0.368241 0.435353 0.499807 0.631725 0.696074 0.726444 0.741485 0.752997 0.755195 0.760334 0.774394 0.8045 0.86873 1 1 1 1
  line L1858 (-93.0015, -42.2716) -> (-95.0015, -34.9516)
  line L1859 (-99.0015, -34.9516) -> (-101.0015, -42.2716)
  line L1860 (-93.0015, -53.6936) -> (-93.0015, -42.2716)
  line L1861 (-101.0015, -53.6936) -> (-101.0015, -42.2716)
  line L1862 (-95.0015, -34.9516) -> (-99.0015, -34.9516)
  line L1863 (-93.0015, -53.6936) -> (-93.0015, -54.7096)
  line L1864 (-101.0015, -53.6936) -> (-101.0015, -54.7096)
  line L1865 (-93.0015, -54.7096) -> (-101.0015, -54.7096)
  line L1866 (-105.1265, -54.7096) -> (-105.3014, -54.7096)
  line L1867 (-105.1265, -54.2016) -> (-105.1265, -54.7096)
  line L1868 (-101.4241, -54.7096) -> (-105.1265, -54.7096)
  line L1869 (-101.4241, -54.7096) -> (-101.0015, -54.7096)
  line L1870 (-93.0015, -54.7096) -> (-92.579, -54.7096)
  line L1871 (-88.8766, -54.7096) -> (-92.579, -54.7096)
  line L1872 (-88.8766, -54.2016) -> (-88.8766, -54.7096)
  line L1873 (-88.7017, -54.7096) -> (-88.8766, -54.7096)
  line L1874 (-105.3014, -54.2016) -> (-105.3014, -54.7096)
  line L1875 (-88.7017, -54.2016) -> (-88.7017, -54.7096)
  line L1876 (-108.0015, -57.8016) -> (-86.0015, -57.8016)
  line L1877 (-108.0015, -90.8016) -> (-86.0015, -90.8016)
  line L1878 (-108.0015, -90.8016) -> (-108.0015, -57.8016)
  line L1879 (-86.0015, -90.8016) -> (-86.0015, -57.8016)
  line L1880 (-106.4, -57.8016) -> (-106.4, -54.8016)
  line L1881 (-104.3, -57.8016) -> (-104.3, -54.8016)
  line L1882 (-98.0515, -57.8016) -> (-98.0515, -54.8016)
  line L1883 (-95.9515, -57.8016) -> (-95.9515, -54.8016)
  line L1884 (-89.7031, -57.8016) -> (-89.7031, -54.8016)
  line L1885 (-87.6031, -57.8016) -> (-87.6031, -54.8016)
  point P0 (0, 0)